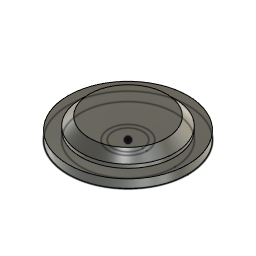
turntable spool polymaker spindle v1 (Autodesk Fusion 360 design; units mm, degrees)
Autodesk Fusion 360 part; units mm, degrees
sketch "Sketch1" plane through (0, 0, 0) normal (0, 0, 1) x (1, 0, 0)
  circle A0 centre (0, 0) radius 27.5
  circle A1 centre (0, 0) radius 35
  circle A2 centre (0, 0) radius 11.1
  circle A3 centre (0, 0) radius 8.6
  dimension "d1" = 55
  dimension "d2" = 70
  dimension "d3" = 22.2
  dimension "d4" = 17.2
  constraint coincident A0.centre A1.centre
  constraint concentric A0 A2
  constraint concentric A2 A3
  measures "d1" diameter of A0
  measures "d2" diameter of A1
  measures "d3" diameter of A2
  measures "d4" diameter of A3
extrude "Extrude1" add sketch "Sketch1" along normal blind 7.1 contours A2
extrude "Extrude2" add sketch "Sketch1" along normal blind 5 from surface at 7.1 contours A2 | A3
extrude "Extrude3" add sketch "Sketch1" along normal blind 5 contours A0 | A1
extrude "Extrude4" add sketch "Sketch1" along normal blind 12.1 contours A0
chamfer "Chamfer1" distance 5 angle 45 1 edges at (-25.639, -9.9444, 12.1)
extrude "Extrude5" cut sketch "Sketch1" along normal blind 7.1 contours A2
equation "d1 = SpoolHoleID"
equation "d2 = SpoolShelfOD"
equation "d3 = BearingOD"
equation "d4 = BearingOD - bearingHolderWallThickness"
equation "BearingOD = 22.20 mm"
equation "bearingHolderWallThickness = 5 mm"
equation "SpoolHoleID = 55 mm"
equation "SpoolShelfOD = 70 mm"
equation "SpoolShelfThickness = 5 mm"
equation "SpoolInsertHeight = 5 mm"
equation "SpoolInsertChamfer = 5 mm"
equation "BearingHeight = 7.10 mm"
equation "d13 = BearingHeight"
equation "d15 = BearingHeight"
equation "d16 = SpoolShelfThickness"
equation "d18 = SpoolShelfThickness"
equation "d20 = SpoolShelfThickness + BearingHeight"
equation "d22 = SpoolInsertChamfer"
equation "d23 = BearingHeight"
